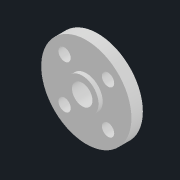
# Autodesk Inventor part: shaftmount
Saved by Autodesk Inventor 2022.2 (Build 262287010, 287A)
## iProperties
Created: 2023-07-21
Part Number: shaftmount
Material: Generic
Document SubType Name: Modeling
Designer: StijnC
Density: 1 g/cm^3
Appearance: Default
Author: StijnC
Autodesk Inventor part; units mm, degrees
ref_plane "YZ Plane" through (0, 0, 0) normal (1, 0, 0) x (0, 1, 0)
ref_plane "XZ Plane" through (0, 0, 0) normal (0, 1, 0) x (-1, 0, 0)
ref_plane "XY Plane" through (0, 0, 0) normal (0, 0, 1) x (1, 0, 0)
sketch "Sketch1" plane through (0, 0, 0) normal (0, 0, 1) x (1, 0, 0)
  circle A0 centre (0, 0) radius 11
  circle A1 centre (0, 0) radius 2.5
  dimension "d0" = 22
  dimension "d1" = 5
  constraints: 2 centre point, 2 coincident
  measures "d0" diameter of A0
  measures "d1" diameter of A1
extrude "Extrusion1" add sketch "Sketch1" along normal mid plane 2.8
sketch "Sketch2" plane through (0, 0, 1.4) normal (0, 0, 1) x (1, 0, 0)
  circle A0 centre (0, 0) radius 7.5 construction
  point P0 (-5.3033, 5.3033)
  point P1 (5.3033, 5.3033)
  point P2 (-5.3033, -5.3033)
  point P3 (5.3033, -5.3033)
  dimension "d4" = 15
  dimension "d5" = 90
  constraints: 3 point on circle, 2 horizontal alignment, 2 vertical alignment, 1 centre point, 1 coincident
  measures "d4" diameter of A0
hole "Hole1" at (-5.3033, 5.3033, 1.4) at (5.3033, 5.3033, 1.4) at (-5.3033, -5.3033, 1.4) at (5.3033, -5.3033, 1.4) direction (0, 0, -1) diameter 3 end through all
sketch "Sketch3" plane through (0, 0, 1.4) normal (0, 0, 1) x (1, 0, 0)
  circle A0 centre (0, 0) radius 4
  circle A1 centre (0, 0) radius 2.5 projected
  dimension "d13" = 8
  constraints: 1 centre point, 1 coincident
  measures "d13" diameter of A0
extrude "Extrusion2" add sketch "Sketch3" along normal blind 1
body "Solid1"
